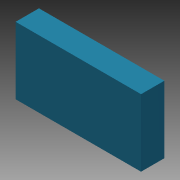
# Autodesk Inventor part: LiPo
Saved by Autodesk Inventor 2013 (Build 170138000, 138)
## iProperties
Created: 2015-07-02
Part Number: LiPo
Material: Aluminum 6061
Document SubType Name: Modeling
Designer: Kyle
Mass: 28.5335 g
Surface Area: 79.5263 cm^2
Volume: 10.529 cm^3
Density: 2.71 g/cm^3
Author: Kyle
Autodesk Inventor part; units mm, degrees
ref_plane "YZ Plane" through (0, 0, 0) normal (1, 0, 0) x (0, 1, 0)
ref_plane "XZ Plane" through (0, 0, 0) normal (0, 1, 0) x (-1, 0, 0)
ref_plane "XY Plane" through (0, 0, 0) normal (0, 0, 1) x (1, 0, 0)
sketch "Sketch1" plane through (0, 0, 0) normal (0, 0, 1) x (1, 0, 0)
  line L0 (0, 0) -> (54.61, 0)
  line L1 (54.61, 0) -> (54.61, 29.21)
  line L2 (54.61, 29.21) -> (0, 29.21)
  line L3 (0, 29.21) -> (0, 0)
  dimension "d0" = 54.61
  dimension "d2" = 29.21
  constraints: 8 end point, 2 parallel, 1 horizontal, 1 perpendicular
  measures "d0" distance of L1.end L2.end
  measures "d2" distance of L2.end L0.start
extrude "Extrusion1" add sketch "Sketch1" along normal blind 10.16
shell "Shell1" thickness 2.667 removed faces 0
body "Solid1"
